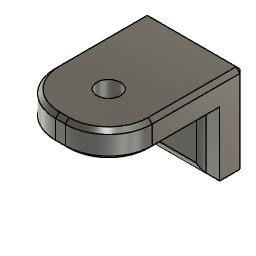
Tube_arm_F695_mount (Autodesk Fusion 360 design; units mm, degrees)
Autodesk Fusion 360 part; units mm, degrees
sketch "sketch 680" plane through (0, 380, 0) normal (0, -1, 0) x (1, 0, 0)
  line L0 (-185.0624, -39) -> (-185.0624, -21)
  line L1 (-185.0624, -21) -> (-205.0624, -21)
  line L2 (-185.0624, -21) -> (-205.0624, -21)
  line L3 (-205.0624, -21) -> (-205.0624, -39)
  line L4 (-205.0624, -39) -> (-185.0624, -39)
extrude "Extrude1" add sketch "sketch 680" along normal blind 7
sketch "sketch 730" plane through (0, 373, 0) normal (0, -1, 0) x (1, 0, 0)
  line L0 (-185.0624, -26.5) -> (-205.0624, -26.5)
  line L1 (-185.0624, -21) -> (-185.0624, -26.5)
  line L2 (-185.0624, -21) -> (-185.0624, -26.5)
  line L3 (-205.0624, -21) -> (-185.0624, -21)
  line L4 (-205.0624, -21) -> (-185.0624, -21)
  line L5 (-205.0624, -26.5) -> (-205.0624, -21)
  line L6 (-205.0624, -26.5) -> (-205.0624, -21)
extrude "Extrude4" add sketch "sketch 730" along normal blind 21
sketch "sketch 715" plane through (0, 373, 0) normal (0, -1, 0) x (1, 0, 0)
  circle A0 centre (-195.0624, -30) radius 1.7
  circle A1 centre (-195.0624, -30) radius 3
extrude "Extrude3" cut sketch "sketch 715" against normal blind 3
sketch "sketch 703" plane through (0, 373, 0) normal (0, -1, 0) x (1, 0, 0)
  circle A0 centre (-195.0624, -30) radius 1.7
extrude "Extrude2" cut sketch "sketch 703" against normal blind 7
sketch "sketch 754" plane through (0, 0, -30.5) normal (0, 0, -1) x (1, 0, 0)
  circle A0 centre (-195.0624, -362) radius 2.425
extrude "Extrude5" cut sketch "sketch 754" against normal blind 10
fillet "Fillet1" radius 9 2 edges at (-185.0624, 352, -23.75) (-205.0624, 352, -23.75)
chamfer "Chamfer1" distance 0.8 angle 45 10 edges at (-205.0624, 370.5, -21) (-202.4264, 354.636, -21) (-195.0624, 352, -21) (-187.6985, 354.636, -21) (-185.0624, 370.5, -21) (-205.0624, 367, -26.5) (-202.4264, 354.636, -26.5) (-195.0624, 352, -26.5) (-187.6985, 354.636, -26.5) (-185.0624, 367, -26.5) 1 faces at (-202.2958, 380, -30)
chamfer "Chamfer2" distance 2 angle 45 3 edges at (-205.0624, 373, -32.75) (-195.0624, 373, -39) (-185.0624, 373, -32.75)
fillet "Fillet2" radius 2 3 edges at (-203.0624, 373, -31.75) (-195.0624, 373, -37) (-187.0624, 373, -31.75)
sketch "Sketch1" plane through (0, 0, -26.5) normal (0, 0, -1) x (1, 0, 0)
  line L0 (-185.8624, -374.2) -> (-185.8624, -361)
  arc A0 (-185.8624, -361) -> (-194.0624, -352.8) centre (-194.0624, -361) ccw
  line L1 (-194.0624, -352.8) -> (-196.0624, -352.8)
  arc A1 (-196.0624, -352.8) -> (-204.2624, -361) centre (-196.0624, -361) ccw
  line L2 (-204.2624, -361) -> (-204.2624, -374.2)
  line L3 (-204.2624, -374.2) -> (-203.6482, -373.5858)
  arc A2 (-202.234, -373) -> (-203.6482, -373.5858) centre (-202.234, -375) ccw
  line L4 (-202.234, -373) -> (-187.8909, -373)
  arc A3 (-186.4766, -373.5858) -> (-187.8909, -373) centre (-187.8909, -375) ccw
  line L5 (-186.4766, -373.5858) -> (-185.8624, -374.2)
  circle A4 centre (-195.0624, -362) radius 2.425
  circle A5 centre (-195.0624, -362) radius 6.25
  dimension "d1" = 12.5
  constraint concentric A4 A5
  measures "d1" diameter of A5
extrude "Extrude6" add sketch "Sketch1" along normal blind 0.2 contours A5
chamfer "Chamfer3" distance 0.2 angle 45 1 edges at (-200.8895, 359.7399, -26.5)
named bodies: "Tube mount"
